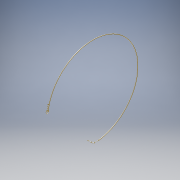
# Autodesk Inventor part: +XPanel_AntennaStowed+Y
Saved by Autodesk Inventor 2018 (Build 220112000, 112)
## iProperties
Created: 2018-07-06
Part Number: +XPanel_AntennaStowed+Y
Material: Titanium
Document SubType Name: Modeling
Designer: Bradley
Density: 4.51 g/cm^3
Appearance: Titanium
Author: Bradley
Autodesk Inventor part; units mm, degrees
ref_plane "XY Plane" through (0, 0, 0) normal (0, 0, 1) x (1, 0, 0)
sketch "Sketch3" plane through (0, 0, 0) normal (0, 1, 0) x (-1, 0, 0)
  circle A0 centre (0, 0) radius 0.2794
  dimension "d7" = 0.5588
  constraints: 1 centre point, 1 coincident
  measures "d7" diameter of A0
sketch "Sketch4" plane through (0, 0, 0) normal (0, 0, 1) x (1, 0, 0)
  line L0 (-4.2178, -1) -> (-1.5, -1)
  line L1 (0, 0) -> (0, 3.5714)
  spline S0 degree 4 poles (-1.5, -1) (-1.2557, -1) (-0.7672, -1) (0, -0.8266) (0, -0.2755) (0, 0) knots 0 0 0 0 0 0.5 1 1 1 1 1
  circle A0 centre (-38.6, -2) radius 39 construction
  dimension "d18" = 78
  dimension "d8" = 1
  dimension "d9" = 1.5
  dimension "d10" = 2.7178
  dimension "d11" = 3.5714
  dimension "d19" = 1
  dimension "d20" = 38.6
  constraints: 4 end point, 2 horizontal, 2 vertical, 5 other
  measures "d8" distance from line of L0 L1.start
  measures "d9" horizontal distance of L0.end L1.start
  measures "d10" distance of L0.start L0.end
  measures "d11" distance of L1.start L1.end
  measures "d19" distance from line of L0 point (-38.6, -2)
  measures "d20" distance from line of L1 point (-38.6, -2)
ref_plane "Work Plane1" through (-38.6, -2, 0) normal (0, 1, 0) x (-1, 0, 0)
sketch "Sketch6" plane through (0.4, -2, 0) normal (0, 1, 0) x (-1, 0, 0)
  line L0 (-2.3178, 38.6) -> (0.4, 38.6)
  point P0 (0.4, 0)
  dimension "d21" = 38.6
  dimension "d22" = 2.7178
  constraints: 2 end point, 1 horizontal, 1 vertical alignment
  measures "d21" distance from line of L0 point (0.4, 0)
  measures "d22" distance of L0.start L0.end
sweep "Sweep3" add profiles "Sketch3" path "Sketch4"
sketch "Sketch7" plane through (0, 3.5714, 0) normal (0, 1, 0) x (1, 0, 0)
  circle A0 centre (0, 0) radius 0.2794 projected
  point P0 (0, 0)
coil "Coil1" sketch "Sketch7" operation add axis through (2.7178, -2, 38.6) along (1, 0, 0) pitch 1.25 turns 0.700941 hand right
sketch "Sketch8" plane through (0.8762, -40.471, 45.0019) normal (0, -0.3033858, -0.9528678) x (-1, 0, 0)
  circle A0 centre (0, 0) radius 0.2794 projected
  point P0 (0.8762, 52.2164)
  point P1 (-0.2794, 0)
  constraints: 1 horizontal alignment
ref_plane "Work Plane2" through (0.8762, -40.471, 45.0019) normal (1, 0, 0) x (0, 1, 0)
sketch "Sketch9" plane through (0.8762, -40.471, 45.0019) normal (1, 0, 0) x (0, 1, 0)
  arc A0 (0, 0) -> (0.2302, -0.8184) centre (0.9864, -0.1642) ccw
  arc A1 (-1.0637, -0.6295) -> (0.2302, -0.8184) centre (-0.5261, -1.4727) ccw
  arc A2 (-1.0637, -0.6295) -> (-0.6146, 0.0508) centre (-1.6013, 0.2137) ccw
  arc A3 (0.2349, 3.9578) -> (-0.6146, 0.0508) centre (38.471, -6.4019) ccw
  circle A4 centre (38.471, -6.4019) radius 39 construction
  circle A5 centre (38.471, -6.4019) radius 39.3073 construction
  point P0 (40.471, -45.0019)
  dimension "d34" = 0.3073
  dimension "d33" = 1
  dimension "d35" = 0.3073
  dimension "d36" = 4
  constraints: 9 point on circle, 4 centre point, 4 equal radius, 3 coincident, 1 tangent, 8 other
  measures "d33" radius of A0
sweep "Sweep4" add profiles "Sketch8" path "Sketch9"
equation "\"d21\" = d20"
equation "\"d22\" = d10"
equation "\"d34\" = 0.55 * d7"
equation "\"d35\" = d34"
body "Solid3"
